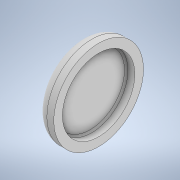
# Autodesk Inventor part: Регулировка
Saved by Autodesk Inventor 2021 (Build 250183000, 183)
## iProperties
Created: 2023-04-26
Part Number: Регулировка
Material: Типовые
Document SubType Name: Modeling
Designer: gdevc
Density: 1 g/cm^3
Appearance: По умолчанию
Author: gdevc
Autodesk Inventor part; units mm, degrees
ref_plane "YZ Plane" through (0, 0, 0) normal (1, 0, 0) x (0, 1, 0)
ref_plane "XZ Plane" through (0, 0, 0) normal (0, 1, 0) x (-1, 0, 0)
ref_plane "XY Plane" through (0, 0, 0) normal (0, 0, 1) x (1, 0, 0)
sketch "Эскиз1" plane through (0, 0, 0) normal (0, 0, 1) x (1, 0, 0)
  line L0 (0, 0) -> (28.3511, 0) construction
  line L1 (0, 20) -> (0, 0)
  line L2 (1, 21) -> (5, 21)
  arc A0 (1, 21) -> (0, 20) centre (1, 20) ccw
  line L3 (5, 26) -> (1, 26)
  arc A1 (1, 26) -> (-5, 20) centre (1, 20) ccw
  line L4 (-5, 20) -> (-5, 0)
  line L5 (-5, 0) -> (3.5853, 0) construction
  line L6 (5, 26) -> (5, 21)
  line L7 (-5, 0) -> (0, 0)
  dimension "d0" = 42
  dimension "d1" = 1
  dimension "d2" = 5
  dimension "d3" = 52
  dimension "d5" = 10
  constraints: 16 end point, 4 point on circle, 2 centre point, 2 horizontal, 2 point on line, 2 tangent, 2 vertical, 1 collinear, 1 other
  measures "d0" diameter of L2 L0
  measures "d1" radius of A0
  measures "d2" distance between parallel lines of L2 L3
  measures "d3" diameter of L3 L0
  measures "d5" distance between parallel lines of L6 L4
revolve "Вращение1" add sketch "Эскиз1" angle 360 about axis through (0, 0, 0) along (1, 0, 0)
